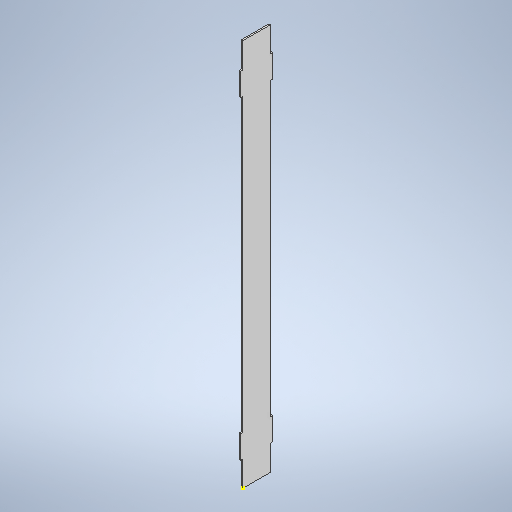
# Autodesk Inventor part: FUNDO CONTRA
Saved by Autodesk Inventor 2025.2 (Build 292293000, 293)
## iProperties
Created: 2025-05-13
Part Number: FUNDO CONTRA
Material: Genérico
Document SubType Name: Modeling
Designer: marce
Density: 1 g/cm^3
Appearance: Padrão
Author: marce
Autodesk Inventor part; units mm, degrees
ref_plane "YZ Plane" through (0, 0, 0) normal (1, 0, 0) x (0, 1, 0)
ref_plane "XZ Plane" through (0, 0, 0) normal (0, 1, 0) x (-1, 0, 0)
ref_plane "XY Plane" through (0, 0, 0) normal (0, 0, 1) x (1, 0, 0)
sketch "Esboço1" plane through (0, 0, 0) normal (1, 0, 0) x (0, 1, 0)
  line L0 (1012, 0) -> (1012, -72)
  line L1 (0, -72) -> (0, 0)
  line L2 (1012, 0) -> (946, 0)
  line L3 (946, 0) -> (946, 6)
  line L4 (946, 6) -> (886, 6)
  line L5 (886, 6) -> (886, 0)
  line L6 (0, 0) -> (66, 0)
  line L7 (66, 0) -> (66, 6)
  line L8 (66, 6) -> (126, 6)
  line L9 (126, 6) -> (126, 0)
  line L10 (126, 0) -> (886, 0)
  line L11 (1012, -72) -> (946, -72)
  line L12 (946, -72) -> (946, -78)
  line L13 (946, -78) -> (886, -78)
  line L14 (886, -78) -> (886, -72)
  line L15 (886, -72) -> (126, -72)
  line L16 (126, -72) -> (126, -78)
  line L17 (126, -78) -> (66, -78)
  line L18 (66, -78) -> (66, -72)
  line L19 (66, -72) -> (0, -72)
  dimension "d1" = 72
  dimension "d2" = 66
  dimension "d3" = 6
  dimension "d4" = 60
  dimension "d7" = 6
  dimension "d8" = 6
  dimension "d9" = 60
  dimension "d10" = 66
  dimension "d11" = 6
  dimension "d12" = 66
  dimension "d13" = 6
  dimension "d14" = 60
  dimension "d17" = 1012
  constraints: 40 end point, 13 perpendicular, 4 point on line, 2 horizontal, 1 parallel, 1 vertical
  measures "d1" distance of L0.start L0.end
  measures "d2" distance of L0.start L2.end
  measures "d3" distance of L2.end L3.end
  measures "d4" distance of L3.end L4.end
  measures "d7" distance of L4.end L5.end
  measures "d8" distance of L8.end L9.end
  measures "d9" distance of L7.end L8.end
  measures "d10" distance of L1.end L6.end
  measures "d11" distance of L11.end L12.end
  measures "d12" distance of L18.end L1.start
  measures "d13" distance of L15.end L16.end
  measures "d14" distance of L16.end L17.end
  measures "d17" distance between parallel lines of L1 L0
extrude "Extrusão1" add sketch "Esboço1" along normal blind 4
sketch "Esboço2" plane through (4, 0, 0) normal (1, 0, 0) x (0, 0, -1)
  point P0 (0, 0)
